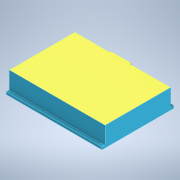
# Autodesk Inventor part: PCB_Tamaño
Saved by Autodesk Inventor 2021 (Build 250183000, 183)
## iProperties
Created: 2022-03-22
Part Number: PCB_Tamaño
Material: Genérico
Document SubType Name: Modeling
Designer: skatl
Density: 1 g/cm^3
Appearance: Turquesa
Author: skatl
Autodesk Inventor part; units mm, degrees
ref_plane "YZ Plane" through (0, 0, 0) normal (1, 0, 0) x (0, 1, 0)
ref_plane "XZ Plane" through (0, 0, 0) normal (0, 1, 0) x (-1, 0, 0)
ref_plane "XY Plane" through (0, 0, 0) normal (0, 0, 1) x (1, 0, 0)
sketch "Boceto1" plane through (0, 0, 0) normal (0, 1, 0) x (-1, 0, 0)
  line L0 (-34, 25.5) -> (34, 25.5)
  line L1 (34, 25.5) -> (34, -25.5)
  line L2 (34, -25.5) -> (-34, -25.5)
  line L3 (-34, -25.5) -> (-34, 25.5)
  line L4 (-34, 25.5) -> (34, -25.5) construction
  line L5 (34, 25.5) -> (-34, -25.5) construction
  point P0 (0, 0)
  dimension "d0" = 68
  dimension "d1" = 51
  constraints: 12 end point, 2 midpoint, 2 parallel, 1 horizontal, 1 perpendicular
  measures "d0" distance of L1.end L2.end
  measures "d1" distance of L0.end L1.end
extrude "Extrusión1" add sketch "Boceto1" along normal blind 14
sketch "Boceto2" plane through (34, 0, 25.5) normal (1, 0, 0) x (0, 0, -1)
  line L0 (51, 0) -> (0, 0) projected
  line L1 (0, 0) -> (2.2, 0)
  line L2 (2.2, 0) -> (2.2, 1.7)
  line L3 (2.2, 1.7) -> (0, 1.7)
  line L4 (0, 1.7) -> (0, 0)
  line L5 (0, 0) -> (0, 14) projected
  line L6 (2.2, 1.7) -> (0, 1.7)
  line L7 (0, 1.7) -> (0, 14)
  line L8 (0, 14) -> (2.2, 14)
  line L9 (2.2, 14) -> (2.2, 1.7)
  line L10 (25.5, -2.8463) -> (25.5, 17.6313)
  line L11 (48.8, 1.7) -> (51, 1.7)
  line L12 (51, 0) -> (51, 14)
  line L13 (51, 14) -> (48.8, 14)
  line L14 (48.8, 14) -> (48.8, 1.7)
  point P0 (25.5, 0)
  dimension "d4" = 2.2
  dimension "d5" = 1.7
  dimension "d8" = 51
  dimension "d9" = 12.3
  dimension "d10" = 46.6
  constraints: 26 end point, 4 parallel, 4 symmetric about line, 2 horizontal, 2 perpendicular, 1 vertical
  measures "d4" distance of L3.end L2.end
  measures "d5" distance of L2.end L1.end
  measures "d8" distance from line of L11.end L4
  measures "d9" distance between parallel lines of L13 L11
  measures "d10" distance between parallel lines of L9 L14
extrude "Extrusión2" cut sketch "Boceto2" against normal through all contours L3 L5 L8 L9 | L14 L13 L12 L11
sketch "Boceto3" plane through (34, 1.7, -23.3) normal (0, 0, -1) x (-1, 0, 0)
  line L0 (68, 12.3) -> (0, 12.3) projected
  line L1 (0, 0) -> (68, 0) projected
  line L2 (0, 12.3) -> (34, 12.3)
  line L3 (34, 12.3) -> (34, 0)
  line L4 (34, 0) -> (0, 0)
  line L5 (0, 0) -> (0, 12.3)
  line L6 (68, 0) -> (68, 12.3) projected
  line L7 (68, 12.3) -> (34, 12.3)
  line L8 (34, 12.3) -> (34, 5.1984)
  line L9 (34, 5.1984) -> (68, 5.1984)
  line L10 (68, 5.1984) -> (68, 12.3)
  line L11 (34, 12.3) -> (23.5366, 12.3)
  line L12 (23.5366, 12.3) -> (28.5366, 12.3)
  line L13 (28.5366, 12.3) -> (43.5366, 12.3)
  line L14 (28.5366, 12.3) -> (43.5366, 12.3)
  line L15 (43.5366, 12.3) -> (43.5366, 5.1984)
  line L16 (43.5366, 5.1984) -> (28.5366, 5.1984)
  line L17 (28.5366, 5.1984) -> (28.5366, 12.3)
  point P0 (34, -1.7)
  point P1 (43.5366, 12.3)
  point P2 (28.5366, 12.3)
  point P3 (34, 5.1984)
  dimension "d11" = 34
  dimension "d12" = 5
  dimension "d13" = 15
  constraints: 30 end point, 6 parallel, 5 point on line, 3 horizontal, 3 perpendicular, 1 midpoint
  measures "d11" distance of L3.end L4.end
  measures "d12" distance of L11.end L12.end
  measures "d13" distance of L12.end L13.end
extrude "Extrusión3" add sketch "Boceto3" along normal blind 1 contours L15 L9 L3 L0 | L3 L16 L17 L0
